REC22-12L Battery_v2 (Autodesk Fusion 360 design; units mm, degrees)
Autodesk Fusion 360 part; units mm, degrees
sketch "Sketch1" plane through (0, 0, 0) normal (0, 0, 1) x (1, 0, 0)
  line L0 (0, 0) -> (183, 0)
  line L1 (183, 0) -> (183, 77)
  line L2 (183, 77) -> (0, 77)
  line L3 (0, 77) -> (0, 0)
  dimension "d1" = 183
  dimension "d2" = 77
  constraint horizontal L0
  constraint vertical L1
  constraint horizontal L2
  constraint vertical L3
  constraint coincident L0.start L3.end
  measures "d1" distance of L0.start L0.end
  measures "d2" distance of L0.start L2.end
extrude "Extrude1" add sketch "Sketch1" along normal blind 169
sketch "Sketch2" plane through (0, 0, 169) normal (0, 0, 1) x (-1, 0, 0)
  line L0 (0, -77) -> (0, 0)
  line L1 (0, 0) -> (-183, 0)
  line L2 (-183, 0) -> (-183, -77)
  line L3 (-183, -77) -> (0, -77)
  line L4 (0, -20) -> (-60, -20)
  line L5 (-60, -20) -> (-60, 0)
  line L6 (-60, 0) -> (0, 0)
  line L7 (0, 0) -> (0, -20)
  line L8 (-183, 0) -> (-123, 0)
  line L9 (-123, 0) -> (-123, -20)
  line L10 (-123, -20) -> (-183, -20)
  line L11 (-183, -20) -> (-183, 0)
  dimension "d5" = 60
  constraint horizontal L4
  constraint vertical L5
  constraint horizontal L6
  constraint vertical L7
  constraint coincident L1 L5.end
  constraint coincident L0 L4.start
  constraint horizontal L8
  constraint vertical L9
  constraint horizontal L10
  constraint vertical L11
  constraint coincident L1.end L2.start
  measures "d5" distance of L1.end L8.end
extrude "Extrude2" cut sketch "Sketch2" against normal blind 20 contours L0 L1 L4 L5 L6 L7 | L1 L2 L8 L9 L10 L11
